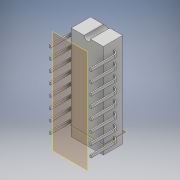
# Autodesk Inventor part: Mikroshema(dokrUGA)
Saved by Autodesk Inventor 2018 (Build 220112000, 112)
## iProperties
Created: 2020-05-16
Part Number: Mikroshema(dokrUGA)
Material: Generic
Document SubType Name: Modeling
Designer: Сергей
Density: 1 g/cm^3
Appearance: Default
Author: Сергей
Autodesk Inventor part; units mm, degrees
ref_plane "YZ Plane" through (0, 0, 0) normal (1, 0, 0) x (0, 1, 0)
ref_plane "XZ Plane" through (0, 0, 0) normal (0, 1, 0) x (-1, 0, 0)
ref_plane "XY Plane" through (0, 0, 0) normal (0, 0, 1) x (1, 0, 0)
sketch "Sketch1" plane through (0, 0, 0) normal (0, 1, 0) x (-1, 0, 0)
  line L0 (-3.75, 11) -> (-3.75, -11)
  line L1 (-3.75, -11) -> (3.75, -11)
  line L2 (3.75, -11) -> (3.75, 11)
  line L3 (3.75, 11) -> (-3.75, -11) construction
  line L4 (-3.75, 11) -> (3.75, -11) construction
  arc A0 (-0.75, 11) -> (0.75, 11) centre (0, 10.9733) ccw
  line L5 (3.75, 11) -> (0.75, 11)
  line L6 (-0.75, 11) -> (-3.75, 11)
  point P0 (0, 0)
  dimension "d0" = 7.5
  dimension "d1" = 22
  constraints: 14 end point, 3 parallel, 2 horizontal, 2 midpoint, 2 perpendicular, 2 point on circle, 1 centre point
  measures "d0" distance of L1.end L0.end
  measures "d1" distance of L0.end L0.start
extrude "Extrusion1" add sketch "Sketch1" along normal mid plane 5
ref_plane "Work Plane1" through (3.75, 2.5, -8.75) normal (0, 0, -1) x (-1, 0, 0)
ref_plane "Work Plane2" through (0, -6.5, 0) normal (0, -1, 0) x (1, 0, 0)
sketch "Sketch4" plane through (3.75, 2.5, -8.75) normal (0, 0, -1) x (-1, 0, 0)
  line L0 (0, 0) -> (0, -5) projected
  line L1 (0, -2.5) -> (0, -2.5)
  line L2 (-1, -3.5) -> (-1, -9)
  arc A0 (0, -2.5) -> (-1, -3.5) centre (0, -3.5) ccw
  point P0 (3.75, -2.5)
  point P1 (-1, -2.5)
  dimension "d10" = 1
  dimension "d11" = 6.5
  dimension "d25" = 1
  constraints: 4 end point, 2 point on circle, 2 point on line, 2 tangent, 1 centre point, 1 horizontal, 1 midpoint, 1 perpendicular
  measures "d10" distance of L1.start point (-1, -2.5)
  measures "d11" distance of point (-1, -2.5) L2.end
  measures "d25" radius of A0
sketch "Sketch6" plane through (0, -6.5, 0) normal (0, -1, 0) x (1, 0, 0)
  line L0 (4.8749, -9.0501) -> (4.6249, -9.0501)
  line L1 (4.6249, -9.0501) -> (4.6249, -8.4501)
  line L2 (4.6249, -8.4501) -> (4.8749, -8.4501)
  line L3 (4.8749, -8.4501) -> (4.8749, -9.0501)
  line L4 (4.8749, -9.0501) -> (4.6249, -8.4501) construction
  line L5 (4.6249, -9.0501) -> (4.8749, -8.4501) construction
  point P0 (0, 0)
  point P1 (4.7499, -8.7501)
  dimension "d18" = 0.25
  dimension "d19" = 0.6
  constraints: 12 end point, 2 midpoint, 2 parallel, 1 horizontal, 1 perpendicular
  measures "d18" distance of L1.end L2.end
  measures "d19" distance of L0.end L1.end
sweep "Sweep2" add profiles "Sketch6" path "Sketch4" path curves L2 A0 L1
pattern_linear "Rectangular Pattern2" count 8 spacing 2.5 along (0, 0, 1) of "Sweep2"
mirror "Mirror2" about plane through (0, 0, 0) normal (1, 0, 0) of "Sweep2", "Rectangular Pattern2"
chamfer "Chamfer1" distance 0.5 angle 45 5 edges at (3.75, 2.5, 0) (0, 2.5, -11) (-3.75, 2.5, 0) (-2.25, 2.5, 11) (2.25, 2.5, 11)
body "Solid1"
